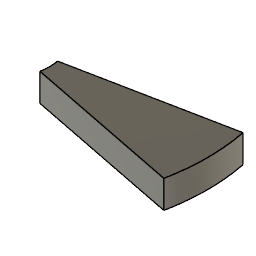
09_SHEX-005_petal_backup (Autodesk Fusion 360 design; units mm, degrees)
part number: 2026-05-30-08-51-12-315
Autodesk Fusion 360 part; units mm, degrees
sketch "Sketch1" plane through (0, 0, 0) normal (0, 0, 1) x (1, 0, 0)
  arc A0 (22.2962, -4.435) -> (22.2962, 4.435) centre (0, 0) ccw
  line L0 (22.2962, 4.435) -> (99.9218, 19.8757)
  arc A1 (99.9218, -19.8757) -> (99.9218, 19.8757) centre (0, 0) ccw
  line L1 (99.9218, -19.8757) -> (22.2962, -4.435)
extrude "Extrude1" add sketch "Sketch1" along normal blind 13.97
named bodies: "SHEX-005_petal"
